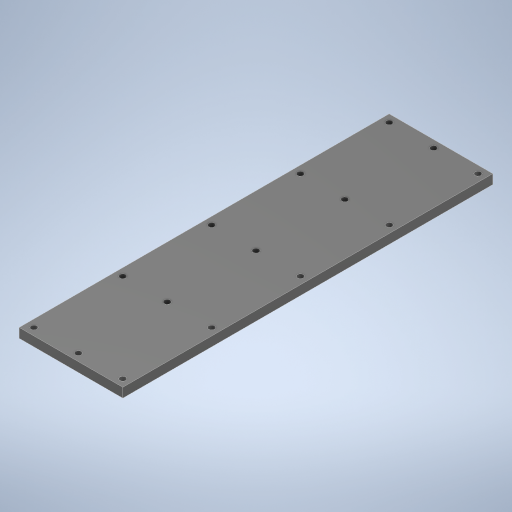
# Autodesk Inventor part: BBM Jig Base
Saved by Autodesk Inventor 2023 (Build 270158000, 158)
## iProperties
Created: 2022-10-25
Part Number: BBM Jig Base
Material: Acetal Resin, Black
Document SubType Name: Modeling
Designer: Caleb
Density: 1.425 g/cm^3
Appearance: Smooth - Black
Author: Caleb
Autodesk Inventor part; units mm, degrees
ref_plane "YZ Plane" through (0, 0, 0) normal (1, 0, 0) x (0, 1, 0)
ref_plane "XZ Plane" through (0, 0, 0) normal (0, 1, 0) x (-1, 0, 0)
ref_plane "XY Plane" through (0, 0, 0) normal (0, 0, 1) x (1, 0, 0)
sketch "Sketch1" plane through (0, 0, 0) normal (0, 1, 0) x (-1, 0, 0)
  line L0 (-17.5, -62.5) -> (17.5, -62.5)
  line L1 (17.5, -62.5) -> (17.5, 62.5)
  line L2 (17.5, 62.5) -> (-17.5, 62.5)
  line L3 (-17.5, 62.5) -> (-17.5, -62.5)
  line L4 (-17.5, -62.5) -> (17.5, 62.5) construction
  line L5 (17.5, -62.5) -> (-17.5, 62.5) construction
  point P0 (0, 0)
  dimension "d0" = 35
  dimension "d1" = 125
  constraints: 12 end point, 2 midpoint, 2 parallel, 1 horizontal, 1 perpendicular
  measures "d0" distance of L2.end L1.end
  measures "d1" distance of L1.end L0.end
extrude "Extrusion1" add sketch "Sketch1" along normal blind 3.175
sketch "Sketch2" plane through (0, 0, 0) normal (0, -1, 0) x (1, 0, 0)
  line L0 (-17.5, 62.5) -> (17.5, 62.5) projected
  line L1 (17.5, 62.5) -> (17.5, -62.5) projected
  line L2 (-17.5, -62.5) -> (-17.5, 62.5) projected
  point P0 (0, 0)
  point P1 (15, 60)
  point P2 (0, 60)
  point P3 (-15, 60)
  point P4 (-15, 30)
  point P5 (0, 30)
  point P6 (15, 30)
  point P7 (-15, 0)
  point P8 (0, 0)
  point P9 (15, 0)
  point P10 (-15, -30)
  point P11 (0, -30)
  point P12 (15, -30)
  point P13 (-15, -60)
  point P14 (0, -60)
  point P15 (15, -60)
  dimension "d4" = 2.5
  dimension "d5" = 2.5
  dimension "d6" = 2.5
  dimension "d9" = 30
  constraints: 2 horizontal alignment, 1 vertical, 1 vertical alignment, 12 other
  measures "d4" distance from line of L0 point (15, 60)
  measures "d5" distance from line of L1 point (15, 60)
  measures "d6" distance from line of L2 point (-15, 60)
  measures "d9" distance of point (-15, 60) point (-15, 30)
hole "Hole1" at (15, 0, 60) at (0, 0, 60) at (-15, 0, 60) at (-15, 0, 30) at (0, 0, 30) at (15, 0, 30) at (-15, 0, 0) at (0, 0, 0) at (15, 0, 0) at (-15, 0, -30) at (0, 0, -30) at (15, 0, -30) at (-15, 0, -60) at (0, 0, -60) at (15, 0, -60) direction (0, 1, 0) diameter 2.057 end through all countersink diameter 3.708 countersink angle 82 clearance for "Flat Head Machine Screw (82)" size "#1" standard "Ansi Unified Screw Threads"
body "Solid1"
